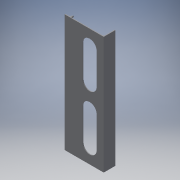
# Autodesk Inventor part: top
Saved by Autodesk Inventor 2019.3 (Build 233278000, 278)
## iProperties
Created: 2019-04-01
Part Number: top
Material: Generic
Document SubType Name: Modeling
Designer: erwin
Density: 1 g/cm^3
Appearance: Default
Author: erwin
Autodesk Inventor part; units mm, degrees
ref_plane "YZ Plane" through (0, 0, 0) normal (1, 0, 0) x (0, 1, 0)
ref_plane "XZ Plane" through (0, 0, 0) normal (0, 1, 0) x (-1, 0, 0)
ref_plane "XY Plane" through (0, 0, 0) normal (0, 0, 1) x (1, 0, 0)
sketch "Sketch1" plane through (0, 0, 0) normal (0, 0, 1) x (1, 0, 0)
  line L0 (44.1114, 5) -> (-5.8886, 5) projected
  line L1 (44.1114, -145) -> (44.1114, 5) projected
  line L2 (-5.8886, -145) -> (44.1114, -145) projected
  line L3 (-5.8886, 5) -> (-5.8886, -145) projected
  arc A0 (17.1114, -55) -> (35.1114, -55) centre (26.1114, -55) ccw projected
  line L4 (35.1114, -55) -> (35.1114, -15) projected
  arc A1 (35.1114, -15) -> (17.1114, -15) centre (26.1114, -15) ccw projected
  line L5 (17.1114, -15) -> (17.1114, -55) projected
  arc A2 (17.1114, -125) -> (35.1114, -125) centre (26.1114, -125) ccw projected
  line L6 (35.1114, -125) -> (35.1114, -85) projected
  arc A3 (35.1114, -85) -> (17.1114, -85) centre (26.1114, -85) ccw projected
  line L7 (17.1114, -85) -> (17.1114, -125) projected
  point P0 (0, 0)
extrude "Extrusion1" add sketch "Sketch1" along normal blind 1 contours L1 L2 L3 L0 | L5 A1 L4 A0 | L7 A3 L6 A2
sketch "Sketch2" plane through (0, 0, 0) normal (0, 0, -1) x (-1, 0, 0)
  line L0 (-44.1114, 5) -> (-43.1114, 5) projected
  line L1 (-43.1114, 5) -> (-43.1114, -145) projected
  line L2 (-43.1114, -145) -> (-44.1114, -145) projected
  line L3 (-44.1114, -145) -> (-44.1114, 5) projected
  point P0 (0, 0)
extrude "Extrusion2" add sketch "Sketch2" along normal blind 14
sketch "Sketch3" plane through (0, 0, 0) normal (0, 0, -1) x (-1, 0, 0)
  point P0 (0, 0)
  point P1 (5.8886, 0)
  point P2 (5.8886, -20)
  point P3 (-3.834, -10)
  point P4 (-3.834, -30)
  point P5 (5.8886, -40)
  point P6 (-3.834, -50)
  point P7 (5.8886, -60)
  point P8 (-3.834, -70)
  point P9 (5.8886, -80)
  point P10 (-3.834, -90)
  point P11 (5.8886, -100)
  point P12 (-3.834, -110)
  point P13 (5.8886, -120)
  point P14 (-3.834, -130)
  point P15 (5.8886, -140)
  constraints: 15 other
sketch "Sketch4" plane through (0, 0, 0) normal (0, 0, -1) x (-1, 0, 0)
  line L0 (5.8886, 0) -> (-4.834, -5) projected
  line L1 (4.4688, 0) -> (-5.0875, 4.4562) projected
  line L2 (-5.0875, -4.4562) -> (4.4688, 0) projected
  line L3 (-4.834, 5) -> (5.8886, 0) projected
  line L4 (0.4688, 0.2102) -> (0.9195, 0)
  line L5 (0.9195, 0) -> (0.4688, -0.2102)
  line L6 (-1.834, 5.2561) -> (1.166, 3.8572)
  line L7 (1.166, -3.8572) -> (-1.834, -5.2561)
  line L8 (0.4688, 1.8652) -> (0.4688, 0.2102)
  line L9 (0.4688, -0.2102) -> (0.4688, -1.8652)
  line L10 (0.4688, 1.8652) -> (4.4688, 0)
  line L11 (4.4688, 0) -> (0.4688, -1.8652)
  line L12 (-1.834, -3.6011) -> (1.166, -2.2022)
  line L13 (1.166, 2.2022) -> (-1.834, 3.6011)
  line L14 (1.166, 2.2022) -> (1.166, 3.8572)
  line L15 (1.166, -2.2022) -> (1.166, -3.8572)
  line L16 (-1.834, -3.6011) -> (-1.834, -5.2561)
  line L17 (-1.834, 5.2561) -> (-1.834, 3.6011)
  line L18 (-1.5309, 2.7977) -> (-1.5309, -2.7977)
  point P0 (0, 0)
  dimension "d4" = 1.5
  dimension "d5" = 1.5
  dimension "d6" = 4
  dimension "d7" = 3
  dimension "d8" = 3
  dimension "d9" = 1.5
  constraints: 30 end point, 6 collinear, 6 point on line, 6 vertical, 3 equal length, 1 parallel
  measures "d4" distance between parallel lines of L1 L4
  measures "d5" distance between parallel lines of L3 L6
  measures "d6" distance from line of L1.start L9
  measures "d7" distance between parallel lines of L15 L16
  measures "d8" distance from line of L0.end L16
  measures "d9" distance between parallel lines of L7 L0
extrude "Extrusion3" add sketch "Sketch4" along normal blind 3 contours L15 L7 L16 L0 | L2 L9 L5 L4 L8 L1 | L17 L6 L14 L3
pattern_sketch "Sketch Driven Pattern1" of "Extrusion3" from (-5.8886, 0, 0) copies at (-5.8886, -20, 0) at (3.834, -10, 0) at (3.834, -30, 0) at (-5.8886, -40, 0) at (3.834, -50, 0) at (-5.8886, -60, 0) at (3.834, -70, 0) at (-5.8886, -80, 0) at (3.834, -90, 0) at (-5.8886, -100, 0) at (3.834, -110, 0) at (-5.8886, -120, 0) at (3.834, -130, 0) at (-5.8886, -140, 0)
fillet "Fillet1" radius 2 1 edges at (43.1114, -70, 0)
sketch "Sketch5" plane through (0, 0, 1) normal (0, 0, 1) x (1, 0, 0)
  arc A0 (17.1114, -55) -> (35.1114, -55) centre (26.1114, -55) ccw projected
  line L0 (17.1114, -55) -> (17.1114, -15) projected
  arc A1 (35.1114, -15) -> (17.1114, -15) centre (26.1114, -15) ccw projected
  line L1 (35.1114, -15) -> (35.1114, -55) projected
  arc A2 (17.1114, -125) -> (35.1114, -125) centre (26.1114, -125) ccw projected
  line L2 (17.1114, -125) -> (17.1114, -85) projected
  arc A3 (35.1114, -85) -> (17.1114, -85) centre (26.1114, -85) ccw projected
  line L3 (35.1114, -85) -> (35.1114, -125) projected
  line L4 (14.5565, -125) -> (14.8101, -125.5438) projected
  line L5 (14.8101, -125.5438) -> (5.2537, -130) projected
  line L6 (5.2537, -130) -> (14.8101, -134.4562) projected
  line L7 (14.8101, -134.4562) -> (14.5565, -135) projected
  line L8 (14.5565, -135) -> (3.834, -130) projected
  line L9 (3.834, -130) -> (14.5565, -125) projected
  line L10 (14.5565, -105) -> (14.8101, -105.5438) projected
  line L11 (14.8101, -105.5438) -> (5.2537, -110) projected
  line L12 (5.2537, -110) -> (14.8101, -114.4562) projected
  line L13 (14.8101, -114.4562) -> (14.5565, -115) projected
  line L14 (14.5565, -115) -> (3.834, -110) projected
  line L15 (3.834, -110) -> (14.5565, -105) projected
  line L16 (14.5565, -85) -> (14.8101, -85.5438) projected
  line L17 (14.8101, -85.5438) -> (5.2537, -90) projected
  line L18 (5.2537, -90) -> (14.8101, -94.4562) projected
  line L19 (14.8101, -94.4562) -> (14.5565, -95) projected
  line L20 (14.5565, -95) -> (3.834, -90) projected
  line L21 (3.834, -90) -> (14.5565, -85) projected
  line L22 (14.5565, -65) -> (14.8101, -65.5438) projected
  line L23 (14.8101, -65.5438) -> (5.2537, -70) projected
  line L24 (5.2537, -70) -> (14.8101, -74.4562) projected
  line L25 (14.8101, -74.4562) -> (14.5565, -75) projected
  line L26 (14.5565, -75) -> (3.834, -70) projected
  line L27 (3.834, -70) -> (14.5565, -65) projected
  line L28 (14.5565, -45) -> (14.8101, -45.5438) projected
  line L29 (14.8101, -45.5438) -> (5.2537, -50) projected
  line L30 (5.2537, -50) -> (14.8101, -54.4562) projected
  line L31 (14.8101, -54.4562) -> (14.5565, -55) projected
  line L32 (14.5565, -55) -> (3.834, -50) projected
  line L33 (3.834, -50) -> (14.5565, -45) projected
  line L34 (14.5565, -25) -> (14.8101, -25.5438) projected
  line L35 (14.8101, -25.5438) -> (5.2537, -30) projected
  line L36 (5.2537, -30) -> (14.8101, -34.4562) projected
  line L37 (14.8101, -34.4562) -> (14.5565, -35) projected
  line L38 (14.5565, -35) -> (3.834, -30) projected
  line L39 (3.834, -30) -> (14.5565, -25) projected
  line L40 (14.5565, -5) -> (14.8101, -5.5438) projected
  line L41 (14.8101, -5.5438) -> (5.2537, -10) projected
  line L42 (5.2537, -10) -> (14.8101, -14.4562) projected
  line L43 (14.8101, -14.4562) -> (14.5565, -15) projected
  line L44 (14.5565, -15) -> (3.834, -10) projected
  line L45 (3.834, -10) -> (14.5565, -5) projected
  line L46 (5.0875, -144.4562) -> (4.834, -145) projected
  line L47 (4.834, -145) -> (41.1114, -145) projected
  line L48 (41.1114, 5) -> (41.1114, -145) projected
  line L49 (41.1114, 5) -> (4.834, 5) projected
  line L50 (4.834, 5) -> (5.0875, 4.4562) projected
  line L51 (5.0875, 4.4562) -> (-4.4688, 0) projected
  line L52 (-4.4688, 0) -> (5.0875, -4.4562) projected
  line L53 (5.0875, -4.4562) -> (4.834, -5) projected
  line L54 (4.834, -5) -> (-5.8886, 0) projected
  line L55 (-5.8886, 0) -> (-5.8886, -20) projected
  line L56 (-5.8886, -20) -> (4.834, -15) projected
  line L57 (4.834, -15) -> (5.0875, -15.5438) projected
  line L58 (5.0875, -15.5438) -> (-4.4688, -20) projected
  line L59 (-4.4688, -20) -> (5.0875, -24.4562) projected
  line L60 (5.0875, -24.4562) -> (4.834, -25) projected
  line L61 (4.834, -25) -> (-5.8886, -20) projected
  line L62 (-5.8886, -20) -> (-5.8886, -40) projected
  line L63 (-5.8886, -40) -> (4.834, -35) projected
  line L64 (4.834, -35) -> (5.0875, -35.5438) projected
  line L65 (5.0875, -35.5438) -> (-4.4688, -40) projected
  line L66 (-4.4688, -40) -> (5.0875, -44.4562) projected
  line L67 (5.0875, -44.4562) -> (4.834, -45) projected
  line L68 (4.834, -45) -> (-5.8886, -40) projected
  line L69 (-5.8886, -40) -> (-5.8886, -60) projected
  line L70 (-5.8886, -60) -> (4.834, -55) projected
  line L71 (4.834, -55) -> (5.0875, -55.5438) projected
  line L72 (5.0875, -55.5438) -> (-4.4688, -60) projected
  line L73 (-4.4688, -60) -> (5.0875, -64.4562) projected
  line L74 (5.0875, -64.4562) -> (4.834, -65) projected
  line L75 (4.834, -65) -> (-5.8886, -60) projected
  line L76 (-5.8886, -60) -> (-5.8886, -80) projected
  line L77 (-5.8886, -80) -> (4.834, -75) projected
  line L78 (4.834, -75) -> (5.0875, -75.5438) projected
  line L79 (5.0875, -75.5438) -> (-4.4688, -80) projected
  line L80 (-4.4688, -80) -> (5.0875, -84.4562) projected
  line L81 (5.0875, -84.4562) -> (4.834, -85) projected
  line L82 (4.834, -85) -> (-5.8886, -80) projected
  line L83 (-5.8886, -80) -> (-5.8886, -100) projected
  line L84 (-5.8886, -100) -> (4.834, -95) projected
  line L85 (4.834, -95) -> (5.0875, -95.5438) projected
  line L86 (5.0875, -95.5438) -> (-4.4688, -100) projected
  line L87 (-4.4688, -100) -> (5.0875, -104.4562) projected
  line L88 (5.0875, -104.4562) -> (4.834, -105) projected
  line L89 (4.834, -105) -> (-5.8886, -100) projected
  line L90 (-5.8886, -100) -> (-5.8886, -120) projected
  line L91 (-5.8886, -120) -> (4.834, -115) projected
  line L92 (4.834, -115) -> (5.0875, -115.5438) projected
  line L93 (5.0875, -115.5438) -> (-4.4688, -120) projected
  line L94 (-4.4688, -120) -> (5.0875, -124.4562) projected
  line L95 (5.0875, -124.4562) -> (4.834, -125) projected
  line L96 (4.834, -125) -> (-5.8886, -120) projected
  line L97 (-5.8886, -120) -> (-5.8886, -140) projected
  line L98 (-5.8886, -140) -> (4.834, -135) projected
  line L99 (4.834, -135) -> (5.0875, -135.5438) projected
  line L100 (5.0875, -135.5438) -> (-4.4688, -140) projected
  line L101 (-4.4688, -140) -> (5.0875, -144.4562) projected
  point P0 (0, 0)
extrude "Extrusion4" cut sketch "Sketch5" against normal through all contours L0 A1 L1 A0 | L2 A3 L3 A2
equation "\"d5\" = d4"
equation "\"d9\" = d4"
body "Solid1"
